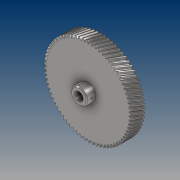
# Autodesk Inventor part: Spur Gear2
Saved by Autodesk Inventor 2021 (Build 250183000, 183)
## iProperties
Created: 2024-03-11
Part Number: Spur Gear2
Material: Stainless Steel, 440C
Document SubType Name: Modeling
Designer: Admin
Categories: <?xml version="1.0" encoding="UTF-16"?> <MemberInstance><Categories><FamilyTemplate><FamilyTemplateParameter ValueType="xs:double" Id="1" ObjectReferenceKey="da_z" ObjectType="kUserParameterObject"/><FamilyTemplateParameter ValueType="xs:double" Id="2" ObjectReferenceKey="da_b" ObjectType="kUserParameterObject"/><FamilyTemplateParameter ValueType="xs:double" Id="3" ObjectReferenceKey="da_beta" ObjectType="kUserParameterObject"/><FamilyTemplateParameter ValueType="xs:double" Id="4" ObjectReferenceKey="da_da" ObjectType="kUserParameterObject"/><FamilyTemplateParameter ValueType="xs:double" Id="5" ObjectReferenceKey="da_aw" ObjectType="kUserParameterObject"/><FamilyTemplateParameter ValueType="xs:string" Id="6" ObjectReferenceKey="EAIAABAAAACIAQAAAAAAAIAAAAAAAAAA" ObjectType="83910656" SubObjectId="SurfaceGeometry"/></FamilyTemplate><ParamToTemplateMap><ParamToTemplate CategoryParameter="//CategoryParameter[@InternalName='046C89C9-8512-4d59-83FE-43B91F4F132A']" TemplateParameter="1"/><ParamToTemplate CategoryParameter="//CategoryParameter[@InternalName='2552DF32-E462-4b46-AEBF-C6C7768E72AC']" TemplateParameter="2"/><ParamToTemplate CategoryParameter="//CategoryParameter[@InternalName='C9EE641D-15FC-4fae-A226-E94C4372FDD7']" TemplateParameter="3"/><ParamToTemplate><ParamToTemplate CategoryParameter="//CategoryParameter[@InternalName='00B6519A-459B-49c7-AD84-2E56D39A5744']" ConstantValue="0.000000"/></ParamToTemplate><ParamToTemplate><ParamToTemplate CategoryParameter="//CategoryParameter[@InternalName='04B31F0E-C7A6-4894-AA32-9629BEFACF47']" ConstantValue="1.000000"/></ParamToTemplate><ParamToTemplate><ParamToTemplate CategoryParameter="//CategoryParameter[@InternalName='43CBEC2E-7847-49e7-A936-2F7889FCB2D9']" ConstantValue="0.250000"/></ParamToTemplate><ParamToTemplate><ParamToTemplate CategoryParameter="//CategoryParameter[@InternalName='B1EFC894-105D-4ebd-86BF-FA20ED196853']" ConstantValue="0.350000"/></ParamToTemplate><ParamToTemplate><ParamToTemplate CategoryParameter="//CategoryParameter[@InternalName='51175063-3D10-4879-93E8-6246FE8B403D']" ConstantValue="2060000000.000000"/></ParamToTemplate><ParamToTemplate><ParamToTemplate CategoryParameter="//CategoryParameter[@InternalName='A3A52E27-4454-46a9-B0BD-C932399B70AF']" ConstantValue="0.300000"/></ParamToTemplate><ParamToTemplate><ParamToTemplate CategoryParameter="//CategoryParameter[@InternalName='91B76062-C214-41d9-B1B9-14D2AB99603D']" ConstantValue="0.125000"/></ParamToTemplate><ParamToTemplate><ParamToTemplate CategoryParameter="//CategoryParameter[@InternalName='374E806E-8B8A-4dda-A9AA-1039D6500AD2']" ConstantValue="8.000000"/></ParamToTemplate><ParamToTemplate><ParamToTemplate CategoryParameter="//CategoryParameter[@InternalName='2D373A89-B862-43d6-8D0B-0CBF12AB9F6C']" ConstantValue="0.349066"/></ParamToTemplate><ParamToTemplate CategoryParameter="//CategoryParameter[@InternalName='37777632-D6A2-4fac-9D53-DB8ACD95C989']" TemplateParameter="4"/><ParamToTemplate CategoryParameter="//CategoryParameter[@InternalName='FD1017F1-B727-4f7e-9707-0F86F1FF9423']" TemplateParameter="5"/><ParamToTemplate><ParamToTemplate CategoryParameter="//CategoryParameter[@InternalName='9E1B4470-B2D3-4ff1-B813-535BB4CDF51A']" ConstantValue="3520000.000000"/></ParamToTemplate><ParamToTemplate><ParamToTemplate CategoryParameter="//CategoryParameter[@InternalName='F8452263-BFF6-458c-9FB1-07C4B99E95CD']" ConstantValue="11400000.000000"/></ParamToTemplate><ParamToTemplate><ParamToTemplate CategoryParameter="//CategoryParameter[@InternalName='3E3BB259-FD49-497f-8171-6EBC954A3479']" ConstantValue="2.000000"/></ParamToTemplate><ParamToTemplate CategoryParameter="//CategoryParameter[@InternalName='27C3BAF2-7550-4e4b-AE2C-0DB134B7D9B7']" TemplateParameter="6"/></ParamToTemplateMap><Category DisplayName="Gear" InternalName="DC85795E-93AB-48d5-8EEE-5A27447B64BD" Mnemonic="Gear"><CategoryParameter DisplayName="z" InternalName="046C89C9-8512-4d59-83FE-43B91F4F132A" Mnemonic="z"/><CategoryParameter DisplayName="b" InternalName="2552DF32-E462-4b46-AEBF-C6C7768E72AC" Mnemonic="b"/><CategoryParameter DisplayName="||b|" InternalName="C9EE641D-15FC-4fae-A226-E94C4372FDD7" Mnemonic="beta"/><CategoryParameter DisplayName="x" InternalName="00B6519A-459B-49c7-AD84-2E56D39A5744" Mnemonic="x"/><CategoryParameter DisplayName="a*" InternalName="04B31F0E-C7A6-4894-AA32-9629BEFACF47" Mnemonic="a"/><CategoryParameter DisplayName="c*" InternalName="43CBEC2E-7847-49e7-A936-2F7889FCB2D9" Mnemonic="c"/><CategoryParameter DisplayName="r|.f|*" InternalName="B1EFC894-105D-4ebd-86BF-FA20ED196853" Mnemonic="rf"/><CategoryParameter DisplayName="E" InternalName="51175063-3D10-4879-93E8-6246FE8B403D" Mnemonic="E"/><CategoryParameter DisplayName="||m|" InternalName="A3A52E27-4454-46a9-B0BD-C932399B70AF" Mnemonic="mi"/><Category DisplayName="SpurGear" InternalName="26C5A22E-A91E-4dfd-A3B3-23CCAFAE1764" Mnemonic="SpurGear"><CategoryParameter DisplayName="m" InternalName="91B76062-C214-41d9-B1B9-14D2AB99603D" Mnemonic="m"/><CategoryParameter DisplayName="P" InternalName="374E806E-8B8A-4dda-A9AA-1039D6500AD2" Mnemonic="PP"/><CategoryParameter DisplayName="||a|" InternalName="2D373A89-B862-43d6-8D0B-0CBF12AB9F6C" Mnemonic="alpha"/><CategoryParameter DisplayName="d|.a|" InternalName="37777632-D6A2-4fac-9D53-DB8ACD95C989" Mnemonic="da"/><CategoryParameter DisplayName="a|.w|" InternalName="FD1017F1-B727-4f7e-9707-0F86F1FF9423" Mnemonic="aw"/><CategoryParameter DisplayName="||s||.Flim|" InternalName="9E1B4470-B2D3-4ff1-B813-535BB4CDF51A" Mnemonic="sFlim"/><CategoryParameter DisplayName="||s||.Hlim|" InternalName="F8452263-BFF6-458c-9FB1-07C4B99E95CD" Mnemonic="sHlim"/><CategoryParameter DisplayName="type" InternalName="3E3BB259-FD49-497f-8171-6EBC954A3479" Mnemonic="type"/><CategoryParameter DisplayName="PitchDiameter" InternalName="27C3BAF2-7550-4e4b-AE2C-0DB134B7D9B7" Mnemonic="IDS_PITCHDIAM"/></Category></Category></Categories></MemberInstance>
Density: 7.75 g/cm^3
Appearance: Semi-Polished
CustomPartVersion: 1
Author: Admin
Autodesk Inventor part; units mm, degrees
sketch "Sketch1" plane through (0, 0, 0) normal (0, 0, 1) x (1, 0, 0)
  circle A0 centre (0, 0) radius 49.138
  dimension "d0" = 98.276
  constraints: 1 centre point
  measures "d0" diameter of A0
extrude "Extrusion1" add sketch "Sketch1" along normal blind 15
ref_plane "Work Plane2" through (0, 0, 7.5) normal (0, 0, 1) x (1, 0, 0)
sketch "Sketch2" plane through (0, 0, 0) normal (0, 0, -1) x (-1, 0, 0)
  circle A0 centre (0, 0) radius 49.138 projected
  circle A1 centre (0, 0) radius 47.888
  dimension "d3" = 95.776
  constraints: 1 centre point, 1 coincident
  measures "d3" diameter of A1
surface extrude "Pitch Diameter" sketch "Sketch2" against normal through all shown no curves A1
ref_plane "Work Plane8" through (0, 0, 0) normal (0.9990482, 0.0436194, 0) x (0, 0, 1)
ref_plane "Work Plane9" through (0, 0, 0) normal (1, 0, 0) x (0, 1, 0)
spur gear teeth "Spur Gear" teeth 72 pitch diameter 95.776 tip diameter 98.276 root diameter 92.651 face width 15 helix angle 20 hand right start plane through (0, 0, 0) normal (0, 0, -1) x (-1, 0, 0)
sketch "Sketch3" plane through (0, 0, 15) normal (0, 0, 1) x (1, 0, 0)
  arc A0 (-13.4677, 47.2564) -> (-14.4954, 46.9513) centre (0, 0) ccw projected
  arc A1 (-17.5351, 45.9028) -> (-18.5323, 45.5093) centre (0, 0) ccw projected
  arc A2 (-21.469, 44.1998) -> (-22.4282, 43.7209) centre (0, 0) ccw projected
  arc A3 (-25.2396, 42.1605) -> (-26.1533, 41.5998) centre (0, 0) ccw projected
  arc A4 (-28.8181, 39.8003) -> (-29.6795, 39.1621) centre (0, 0) ccw projected
  arc A5 (-32.1773, 37.1371) -> (-32.9797, 36.4264) centre (0, 0) ccw projected
  arc A6 (-35.2915, 34.1914) -> (-36.029, 33.4134) centre (0, 0) ccw projected
  arc A7 (-38.1372, 30.9854) -> (-38.8041, 30.1461) centre (0, 0) ccw projected
  arc A8 (-40.6926, 27.5436) -> (-41.2838, 26.6494) centre (0, 0) ccw projected
  arc A9 (-42.9384, 23.8922) -> (-43.4494, 22.9498) centre (0, 0) ccw projected
  arc A10 (-44.8573, 20.059) -> (-45.2842, 19.0756) centre (0, 0) ccw projected
  arc A11 (-46.4349, 16.0731) -> (-46.7745, 15.0563) centre (0, 0) ccw projected
  arc A12 (-47.6591, 11.9648) -> (-47.9087, 10.9223) centre (0, 0) ccw projected
  arc A13 (-48.5205, 7.7656) -> (-48.6784, 6.7052) centre (0, 0) ccw projected
  arc A14 (-49.0127, 3.5072) -> (-49.0775, 2.4371) centre (0, 0) ccw projected
  arc A15 (-49.1318, -0.7779) -> (-49.1032, -1.8495) centre (0, 0) ccw projected
  arc A16 (-48.8771, -5.0571) -> (-48.7551, -6.1221) centre (0, 0) ccw projected
  arc A17 (-48.2503, -9.2978) -> (-48.036, -10.3481) centre (0, 0) ccw projected
  arc A18 (-47.2564, -13.4677) -> (-46.9513, -14.4954) centre (0, 0) ccw projected
  arc A19 (-45.9028, -17.5351) -> (-45.5093, -18.5323) centre (0, 0) ccw projected
  arc A20 (-44.1998, -21.469) -> (-43.7209, -22.4282) centre (0, 0) ccw projected
  arc A21 (-42.1605, -25.2396) -> (-41.5998, -26.1533) centre (0, 0) ccw projected
  arc A22 (-39.8003, -28.8181) -> (-39.1621, -29.6795) centre (0, 0) ccw projected
  arc A23 (-37.1371, -32.1773) -> (-36.4264, -32.9797) centre (0, 0) ccw projected
  arc A24 (-34.1914, -35.2915) -> (-33.4134, -36.029) centre (0, 0) ccw projected
  arc A25 (-30.9854, -38.1372) -> (-30.1461, -38.8041) centre (0, 0) ccw projected
  arc A26 (-27.5436, -40.6926) -> (-26.6494, -41.2838) centre (0, 0) ccw projected
  arc A27 (-23.8922, -42.9384) -> (-22.9498, -43.4494) centre (0, 0) ccw projected
  arc A28 (-20.059, -44.8573) -> (-19.0756, -45.2842) centre (0, 0) ccw projected
  arc A29 (-16.0731, -46.4349) -> (-15.0563, -46.7745) centre (0, 0) ccw projected
  arc A30 (-11.9648, -47.6591) -> (-10.9223, -47.9087) centre (0, 0) ccw projected
  arc A31 (-7.7656, -48.5205) -> (-6.7052, -48.6784) centre (0, 0) ccw projected
  arc A32 (-3.5072, -49.0127) -> (-2.4371, -49.0775) centre (0, 0) ccw projected
  arc A33 (0.7779, -49.1318) -> (1.8495, -49.1032) centre (0, 0) ccw projected
  arc A34 (5.0571, -48.8771) -> (6.1221, -48.7551) centre (0, 0) ccw projected
  arc A35 (9.2978, -48.2503) -> (10.3481, -48.036) centre (0, 0) ccw projected
  arc A36 (13.4677, -47.2564) -> (14.4954, -46.9513) centre (0, 0) ccw projected
  arc A37 (17.5351, -45.9028) -> (18.5323, -45.5093) centre (0, 0) ccw projected
  arc A38 (21.469, -44.1998) -> (22.4282, -43.7209) centre (0, 0) ccw projected
  arc A39 (25.2396, -42.1605) -> (26.1533, -41.5998) centre (0, 0) ccw projected
  arc A40 (28.8181, -39.8003) -> (29.6795, -39.1621) centre (0, 0) ccw projected
  arc A41 (32.1773, -37.1371) -> (32.9797, -36.4264) centre (0, 0) ccw projected
  arc A42 (35.2915, -34.1914) -> (36.029, -33.4134) centre (0, 0) ccw projected
  arc A43 (38.1372, -30.9854) -> (38.8041, -30.1461) centre (0, 0) ccw projected
  arc A44 (40.6926, -27.5436) -> (41.2838, -26.6494) centre (0, 0) ccw projected
  arc A45 (42.9384, -23.8922) -> (43.4494, -22.9498) centre (0, 0) ccw projected
  arc A46 (44.8573, -20.059) -> (45.2842, -19.0756) centre (0, 0) ccw projected
  arc A47 (46.4349, -16.0731) -> (46.7745, -15.0563) centre (0, 0) ccw projected
  arc A48 (47.6591, -11.9648) -> (47.9087, -10.9223) centre (0, 0) ccw projected
  arc A49 (48.5205, -7.7656) -> (48.6784, -6.7052) centre (0, 0) ccw projected
  arc A50 (49.0127, -3.5072) -> (49.0775, -2.4371) centre (0, 0) ccw projected
  arc A51 (49.1318, 0.7779) -> (49.1032, 1.8495) centre (0, 0) ccw projected
  arc A52 (48.8771, 5.0571) -> (48.7551, 6.1221) centre (0, 0) ccw projected
  arc A53 (48.2503, 9.2978) -> (48.036, 10.3481) centre (0, 0) ccw projected
  arc A54 (47.2564, 13.4677) -> (46.9513, 14.4954) centre (0, 0) ccw projected
  arc A55 (45.9028, 17.5351) -> (45.5093, 18.5323) centre (0, 0) ccw projected
  arc A56 (44.1998, 21.469) -> (43.7209, 22.4282) centre (0, 0) ccw projected
  arc A57 (42.1605, 25.2396) -> (41.5998, 26.1533) centre (0, 0) ccw projected
  arc A58 (39.8003, 28.8181) -> (39.1621, 29.6795) centre (0, 0) ccw projected
  arc A59 (37.1371, 32.1773) -> (36.4264, 32.9797) centre (0, 0) ccw projected
  arc A60 (34.1914, 35.2915) -> (33.4134, 36.029) centre (0, 0) ccw projected
  arc A61 (30.9854, 38.1372) -> (30.1461, 38.8041) centre (0, 0) ccw projected
  arc A62 (27.5436, 40.6926) -> (26.6494, 41.2838) centre (0, 0) ccw projected
  arc A63 (23.8922, 42.9384) -> (22.9498, 43.4494) centre (0, 0) ccw projected
  arc A64 (20.059, 44.8573) -> (19.0756, 45.2842) centre (0, 0) ccw projected
  arc A65 (16.0731, 46.4349) -> (15.0563, 46.7745) centre (0, 0) ccw projected
  arc A66 (11.9648, 47.6591) -> (10.9223, 47.9087) centre (0, 0) ccw projected
  arc A67 (7.7656, 48.5205) -> (6.7052, 48.6784) centre (0, 0) ccw projected
  arc A68 (3.5072, 49.0127) -> (2.4371, 49.0775) centre (0, 0) ccw projected
  arc A69 (-0.7779, 49.1318) -> (-1.8495, 49.1032) centre (0, 0) ccw projected
  arc A70 (-5.0571, 48.8771) -> (-6.1221, 48.7551) centre (0, 0) ccw projected
  arc A71 (-9.2978, 48.2503) -> (-10.3481, 48.036) centre (0, 0) ccw projected
  circle A72 centre (0, 0) radius 5
  circle A73 centre (0, 0) radius 9
  dimension "d49" = 10
  dimension "d50" = 4
  constraints: 2 centre point, 1 coincident, 216 other
  measures "d49" diameter of A72
  measures "d50" radial gap between concentric circles of A72 A73
extrude "Extrusion2" cut sketch "Sketch3" against normal blind 22 contours A72
extrude "Extrusion3" add sketch "Sketch3" along normal blind 10
chamfer "Chamfer1" distance 1 angle 45 1 edges at (-9, 0, 25)
sketch "Sketch4" plane through (0, 0, 0) normal (0, 1, 0) x (-1, 0, 0)
  line L0 (-9, 15) -> (9, 15) projected
  line L1 (9, 24) -> (-9, 24) projected
  circle A0 centre (0, 19.5) radius 1.25
  line L2 (9, 24) -> (-9, 24) projected
  line L3 (0, 24) -> (0, 15)
  point P0 (0, 0)
  dimension "d58" = 2.5
  constraints: 3 midpoint, 2 end point, 1 centre point
  measures "d58" diameter of A0
extrude "Extrusion4" cut sketch "Sketch4" against normal blind 15
pattern_circular "Circular Pattern1" count 2 over 90 about axis through (0, 0, 15) along (0, 0, 1) of "Extrusion4"
equation "\"d0\" = da_da"
equation "\"d1\" = da_b"
equation "\"d3\" = da_d"
equation "\"d16\" = da_aw"
equation "\"d43\" = da_aw"
equation "\"d46\" = da_aw"
equation "\"da_da\" = 98.276"
equation "\"da_b\" = 15"
equation "\"da_d\" = 95.776"
equation "\"da_aw\" = 59.86"
body "Solid1"
body "Srf1"
